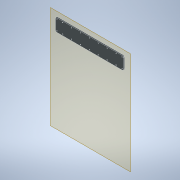
# Autodesk Inventor part: Крышка картера 3
Saved by Autodesk Inventor 2021 (Build 250183000, 183)
## iProperties
Created: 2020-12-12
Part Number: Крышка картера 3
Material: Чугун, серый
Document SubType Name: Modeling
Designer: Тимоха
Mass: 6605.63 g
Surface Area: 2059.71 cm^2
Volume: 923.865 cm^3
Density: 7.15 g/cm^3
Appearance: Чугун серый
Author: Тимоха
Autodesk Inventor part; units mm, degrees
ref_plane "YZ Plane" through (0, 0, 0) normal (1, 0, 0) x (0, 1, 0)
ref_plane "XZ Plane" through (0, 0, 0) normal (0, 1, 0) x (-1, 0, 0)
ref_plane "XY Plane" through (0, 0, 0) normal (0, 0, 1) x (1, 0, 0)
ref_plane "РабПлоскость1" through (0, 0, 0) normal (0, 0, 1) x (1, 0, 0)
sketch "Эскиз1" plane through (0, 0, 0) normal (0, 0, 1) x (1, 0, 0)
  circle A0 centre (340, 472) radius 4 projected
  circle A1 centre (340, 367) radius 4 projected
  circle A2 centre (340, 322.8) radius 4 projected
  circle A3 centre (340, 218.5) radius 4 projected
  circle A4 centre (340, 114.2) radius 4 projected
  circle A5 centre (340, 9.9) radius 4 projected
  circle A6 centre (340, -94.4) radius 4 projected
  circle A7 centre (340, -198.7) radius 4 projected
  circle A8 centre (340, -303) radius 4 projected
  circle A9 centre (340, -347) radius 4 projected
  circle A10 centre (340, -407) radius 4 projected
  circle A11 centre (340, -467) radius 4 projected
  circle A12 centre (278, 472) radius 4 projected
  circle A13 centre (185, 472) radius 4 projected
  circle A14 centre (92, 472) radius 4 projected
  circle A15 centre (-1, 472) radius 4 projected
  circle A16 centre (-94, 472) radius 4 projected
  circle A17 centre (-187, 472) radius 4 projected
  circle A18 centre (-280, 472) radius 4 projected
  circle A19 centre (-340, 472) radius 4 projected
  circle A20 centre (-340, 367) radius 4 projected
  circle A21 centre (-340, 322.8) radius 4 projected
  circle A22 centre (-340, 218.5) radius 4 projected
  circle A23 centre (-340, 114.2) radius 4 projected
  circle A24 centre (-340, 9.9) radius 4 projected
  circle A25 centre (-340, -94.4) radius 4 projected
  circle A26 centre (-340, -198.7) radius 4 projected
  circle A27 centre (-340, -303) radius 4 projected
  circle A28 centre (-340, -347) radius 4 projected
  circle A29 centre (-340, -407) radius 4 projected
  circle A30 centre (-340, -467) radius 4 projected
  line L0 (165, -460) -> (165, -485) projected
  line L1 (185, -485) -> (165, -485) projected
  line L2 (185, -475) -> (185, -485) projected
  line L3 (185, -475) -> (380, -475) projected
  line L4 (380, -475) -> (380, 475) projected
  line L5 (380, 475) -> (350, 475) projected
  line L6 (350, 475) -> (350, 485) projected
  line L7 (-350, 485) -> (350, 485) projected
  line L8 (-350, 475) -> (-350, 485) projected
  line L9 (-350, 475) -> (-380, 475) projected
  line L10 (-380, 475) -> (-380, -475) projected
  line L11 (-380, -475) -> (-185, -475) projected
  line L12 (-185, -475) -> (-185, -485) projected
  line L13 (-165, -485) -> (-185, -485) projected
  line L14 (-165, -485) -> (-165, -460) projected
  line L15 (-165, -460) -> (-330, -460) projected
  line L16 (-330, 460) -> (-330, -460) projected
  line L17 (-330, 460) -> (330, 460) projected
  line L18 (330, -460) -> (330, 460) projected
  line L19 (330, -460) -> (165, -460) projected
  circle A31 centre (278, 367) radius 4 projected
  circle A32 centre (185, 367) radius 4 projected
  circle A33 centre (92, 367) radius 4 projected
  circle A34 centre (-1, 367) radius 4 projected
  circle A35 centre (-94, 367) radius 4 projected
  circle A36 centre (-187, 367) radius 4 projected
  circle A37 centre (-280, 367) radius 4 projected
  circle A38 centre (278, 323) radius 4 projected
  circle A39 centre (185, 323) radius 4 projected
  circle A40 centre (92, 323) radius 4 projected
  circle A41 centre (-1, 323) radius 4 projected
  circle A42 centre (-94, 323) radius 4 projected
  circle A43 centre (-187, 323) radius 4 projected
  circle A44 centre (-280, 323) radius 4 projected
  line L20 (-330, 379) -> (-330, 311) projected
  line L21 (-330, 311) -> (330, 311) projected
  line L22 (330, 379) -> (330, 311) projected
  line L23 (-330, 379) -> (330, 379) projected
  circle A45 centre (340, 367) radius 14
  circle A46 centre (-340, 367) radius 14
  circle A47 centre (-340, 472) radius 14
  circle A48 centre (340, 472) radius 14
  line L24 (354, 472) -> (354, 367)
  line L25 (340, 353) -> (-340, 353)
  line L26 (-354, 367) -> (-354, 472)
  point P0 (0, 0)
  point P1 (353.6748, 475)
  point P2 (350, 481.798)
  point P3 (345.1962, 485)
  point P4 (-345.1962, 485)
  point P5 (-350, 481.798)
  point P6 (-353.6748, 475)
  dimension "d0" = 10
  dimension "d1" = 10
  dimension "d2" = 10
  dimension "d3" = 10
  constraints: 6 end point, 4 point on circle, 2 centre point, 2 vertical, 1 perpendicular, 1 tangent, 6 other
  measures "d0" radial gap between concentric circles of A1 A45
  measures "d1" radial gap between concentric circles of A20 A46
extrude "Выдавливание1" add sketch "Эскиз1" along normal blind 10 contours L25 L16 A46 L23 L18 A45 | L18 A45 L25 | A45 L18 | L18 A45 | L25 A46 L16 | L18 L17 L16 A46 L26 A47 L7 A48 L24 A45 | A46 L16 | L16 A46 | A48 L7 L6 L5 | L23 L16 L17 L18 | A48 L7 L6 | A47 L9 L8 L7 | A47 L8 L7
